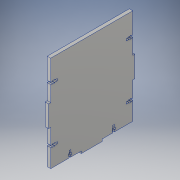
# Autodesk Inventor part: Hopper Wall
Saved by Autodesk Inventor 2018 (Build 220112000, 112)
## iProperties
Created: 2013-10-08
Part Number: Hopper Wall
Material: Aluminum 6061
Document SubType Name: Modeling
Designer: Gabriel Smolnycki
Mass: 428.036 g
Surface Area: 579.08 cm^2
Volume: 158.532 cm^3
Density: 2.7 g/cm^3
Appearance: Aluminum - Flat
Sending System: SolidWorks 2017
Last Author: Gabriel Smolnycki
Last Saved: 2017-09-14
Author: Gabriel Smolnycki
Autodesk Inventor part; units mm, degrees
ref_plane "XZ Plane" through (0, 0, 0) normal (0, 1, 0) x (-1, 0, 0)
ref_plane "XY Plane" through (0, 0, 0) normal (0, 0, 1) x (1, 0, 0)
ref_plane "Work Plane1" through (-6, 0, 0) normal (1, 0, 0) x (0, 1, 0)
sketch "Sketch1" plane through (-6, 0, 0) normal (1, 0, 0) x (0, 1, 0)
  line L0 (-109.5, 75) -> (-138.25, 75)
  line L1 (0, -75) -> (0, 75)
  line L2 (-109.5, 79) -> (-109.5, 75)
  line L3 (-38.25, -75) -> (0, -75)
  line L4 (-138.25, -75) -> (-138.25, -72)
  line L5 (-70.5, 79) -> (-109.5, 79)
  line L6 (-38.25, -75) -> (-38.25, -72)
  line L7 (-138.25, -72) -> (-137.25, -72)
  line L8 (-70.5, 75) -> (-70.5, 79)
  line L9 (-38.25, -72) -> (-37.25, -72)
  line L10 (-137.25, -72) -> (-137.25, -68)
  line L11 (-175, 38.5) -> (-172, 38.5)
  line L12 (-37.25, -72) -> (-37.25, -68)
  line L13 (-137.25, -68) -> (-138.25, -68)
  line L14 (-141.75, 75) -> (-175, 75)
  line L15 (-41.75, 75) -> (-41.75, 72)
  line L16 (-37.25, -68) -> (-38.25, -68)
  line L17 (-138.25, -68) -> (-138.25, -63)
  line L18 (-172, 38.5) -> (-172, 37.25)
  line L19 (-179, -19) -> (-175, -19)
  line L20 (-141.75, 75) -> (-141.75, 72)
  line L21 (-41.75, 72) -> (-42.75, 72)
  line L22 (-38.25, -68) -> (-38.25, -63)
  line L23 (-138.25, -63) -> (-141.75, -63)
  line L24 (-172, 37.25) -> (-168, 37.25)
  line L25 (-175, -75) -> (-141.75, -75)
  line L26 (-179, 19) -> (-179, -19)
  line L27 (-141.75, 72) -> (-142.75, 72)
  line L28 (-42.75, 72) -> (-42.75, 68)
  line L29 (-38.25, -63) -> (-41.75, -63)
  line L30 (-141.75, -63) -> (-141.75, -68)
  line L31 (-172, -42.75) -> (-168, -42.75)
  line L32 (-168, 37.25) -> (-168, 38.5)
  line L33 (-175, 19) -> (-179, 19)
  line L34 (-142.75, 72) -> (-142.75, 68)
  line L35 (-42.75, 68) -> (-41.75, 68)
  line L36 (-41.75, -63) -> (-41.75, -68)
  line L37 (-141.75, -68) -> (-142.75, -68)
  line L38 (-175, -41.5) -> (-172, -41.5)
  line L39 (-168, -42.75) -> (-168, -41.5)
  line L40 (-168, 38.5) -> (-163, 38.5)
  line L41 (-175, 38.5) -> (-175, 19)
  line L42 (-142.75, 68) -> (-141.75, 68)
  line L43 (-41.75, 68) -> (-41.75, 63)
  line L44 (-41.75, -68) -> (-42.75, -68)
  line L45 (-142.75, -68) -> (-142.75, -72)
  line L46 (-168, -41.5) -> (-163, -41.5)
  line L47 (-163, 38.5) -> (-163, 41.5)
  line L48 (-141.75, 68) -> (-141.75, 63)
  line L49 (-41.75, 63) -> (-38.25, 63)
  line L50 (-42.75, -68) -> (-42.75, -72)
  line L51 (-142.75, -72) -> (-141.75, -72)
  line L52 (-163, -41.5) -> (-163, -38.5)
  line L53 (-163, 41.5) -> (-168, 41.5)
  line L54 (0, 75) -> (-38.25, 75)
  line L55 (-163, -38.5) -> (-168, -38.5)
  line L56 (-168, 41.5) -> (-168, 42.75)
  line L57 (-138.25, -75) -> (-109.5, -75)
  line L58 (-141.75, 63) -> (-138.25, 63)
  line L59 (-38.25, 63) -> (-38.25, 68)
  line L60 (-42.75, -72) -> (-41.75, -72)
  line L61 (-141.75, -72) -> (-141.75, -75)
  line L62 (-168, -38.5) -> (-168, -37.25)
  line L63 (-168, 42.75) -> (-172, 42.75)
  line L64 (-172, -41.5) -> (-172, -42.75)
  line L65 (-138.25, 63) -> (-138.25, 68)
  line L66 (-38.25, 68) -> (-37.25, 68)
  line L67 (-41.75, -72) -> (-41.75, -75)
  line L68 (-168, -37.25) -> (-172, -37.25)
  line L69 (-172, 42.75) -> (-172, 41.5)
  line L70 (-138.25, 68) -> (-137.25, 68)
  line L71 (-37.25, 68) -> (-37.25, 72)
  line L72 (-70.5, -75) -> (-41.75, -75)
  line L73 (-175, -41.5) -> (-175, -75)
  line L74 (-172, -37.25) -> (-172, -38.5)
  line L75 (-172, 41.5) -> (-175, 41.5)
  line L76 (-137.25, 68) -> (-137.25, 72)
  line L77 (-37.25, 72) -> (-38.25, 72)
  line L78 (-70.5, -79) -> (-70.5, -75)
  line L79 (-172, -38.5) -> (-175, -38.5)
  line L80 (-175, 75) -> (-175, 41.5)
  line L81 (-41.75, 75) -> (-70.5, 75)
  line L82 (-137.25, 72) -> (-138.25, 72)
  line L83 (-38.25, 72) -> (-38.25, 75)
  line L84 (-109.5, -79) -> (-70.5, -79)
  line L85 (-175, -19) -> (-175, -38.5)
  line L86 (-138.25, 72) -> (-138.25, 75)
  line L87 (-109.5, -75) -> (-109.5, -79)
  constraints: 176 end point, 62 equal length, 44 horizontal, 44 vertical, 11 collinear
extrude "Extrusion1" add sketch "Sketch1" along normal blind 6.35
body "Solid3"
